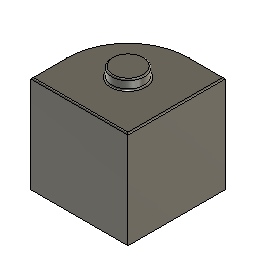
learn1 (Autodesk Fusion 360 design; units mm, degrees)
Autodesk Fusion 360 part; units mm, degrees
sketch "Sketch1" plane through (0, 0, 0) normal (0, 0, 1) x (1, 0, 0) in component "part 1"
  line L0 (0, 0) -> (15, 0)
  line L1 (15, 0) -> (15, 15)
  line L2 (15, 15) -> (0, 15)
  line L3 (0, 15) -> (0, 0)
  constraint horizontal L0
  constraint vertical L1
  constraint horizontal L2
  constraint vertical L3
  constraint coincident L0.start L3.end
extrude "Extrude1" add sketch "Sketch1" along normal blind 15 in component "part 1"
sketch "Sketch2" plane through (0, 0, 15) normal (0, 0, 1) x (-1, 0, 0) in component "part 1"
  line L0 (0, -15) -> (0, 0)
  line L1 (0, 0) -> (-15, 0)
  line L2 (-15, 0) -> (-15, -15)
  line L3 (-15, -15) -> (0, -15)
  circle A0 centre (-7.4741, -7.5439) radius 2.5
  dimension "d3" = 5
  measures "d3" diameter of A0
extrude "Extrude2" add sketch "Sketch2" along normal blind 1 contours A0 in component "part 1"
extrude "Extrude3" add 1 faces at (7.6595, 6.8049, 16) along direction (0, 0, 1) blind 0.5 in component "part 1"
shell "Shell1" thickness 1.4 removed faces 1 at (5, 10, 0) in component "part 1"
fillet "Fillet1" radius 0.2 1 edges at (9.8049, 8.448, 16.5) in component "part 1"
fillet "Fillet2" radius 0.2 1 faces at (7.5536, 1.6836, 15) in component "part 1"
fillet "Fillet3" radius 9.5 2 edges at (0, 15, 7.4) (0.0586, 14.9414, 14.9414) in component "part 1"
component "part 1" placed x (1, 0, 0) y (0, 1, 0) z (0, 0, 1) at (0, 0, 0)
